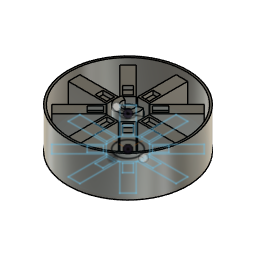
Pill Organiser Archive (Autodesk Fusion 360 design; units mm, degrees)
Autodesk Fusion 360 part; units mm, degrees
note: some values were not read from the file. Set by a fixed rule: which sketch regions a step uses.
sketch "Pill Organiser" plane through (0, 0, 0) normal (0, 0, 1) x (1, 0, 0)
  circle A0 centre (0, 0) radius 150
  dimension "d9" = 300
  constraint coincident A0.centre origin
  measures "d9" diameter of A0
extrude "Extrude2" add sketch "Pill Organiser" along normal blind 30
shell "Shell2" thickness 5 outward yes removed faces 1 at (37.2111, 41.4608, 30)
sketch "Compartment Mounts" plane through (0, 0, 0) normal (0, 0, 1) x (-1, 0, 0)
  circle A0 centre (0, 0) radius 150
  circle A1 centre (0, 0) radius 30
  line L0 (15, -140) -> (-15, -140)
  line L1 (-15, -140) -> (-15, -40)
  line L2 (-15, -40) -> (15, -40)
  line L3 (15, -40) -> (15, -140)
  line L4 (0, -40) -> (0, 0) construction
  line L5 (0, 0) -> (0, 40) construction
  line L6 (-15, 40) -> (-15, 140)
  line L7 (15, 40) -> (-15, 40)
  line L8 (15, 140) -> (15, 40)
  line L9 (-15, 140) -> (15, 140)
  line L10 (140, 15) -> (140, -15)
  line L11 (140, -15) -> (40, -15)
  line L12 (40, -15) -> (40, 15)
  line L13 (40, 15) -> (140, 15)
  line L14 (0, 0) -> (40, 0) construction
  line L15 (0, 0) -> (-40, 0) construction
  line L16 (-140, 15) -> (-40, 15)
  line L17 (-40, 15) -> (-40, -15)
  line L18 (-140, -15) -> (-140, 15)
  line L19 (-40, -15) -> (-140, -15)
  line L20 (10, -45) -> (-10, -45)
  line L21 (-10, -45) -> (-10, -75)
  line L22 (-10, -75) -> (10, -75)
  line L23 (10, -75) -> (10, -45)
  line L24 (-45, -10) -> (-75, -10)
  line L25 (-75, -10) -> (-75, 10)
  line L26 (-75, 10) -> (-45, 10)
  line L27 (-45, 10) -> (-45, -10)
  line L28 (10, 45) -> (-10, 45)
  line L29 (-10, 45) -> (-10, 75)
  line L30 (-10, 75) -> (10, 75)
  line L31 (10, 75) -> (10, 45)
  line L32 (75, -10) -> (45, -10)
  line L33 (45, -10) -> (45, 10)
  line L34 (45, 10) -> (75, 10)
  line L35 (75, 10) -> (75, -10)
  line L36 (-109.6016, -88.3883) -> (-38.8909, -17.6777)
  line L37 (-38.8909, -17.6777) -> (-17.6777, -38.8909)
  line L38 (-17.6777, -38.8909) -> (-88.3883, -109.6016)
  line L39 (-88.3883, -109.6016) -> (-109.6016, -88.3883)
  line L40 (-38.8909, -24.7487) -> (-24.7487, -38.8909)
  line L41 (-24.7487, -38.8909) -> (-45.9619, -60.1041)
  line L42 (-60.1041, -45.9619) -> (-38.8909, -24.7487)
  line L43 (-45.9619, -60.1041) -> (-60.1041, -45.9619)
  line L44 (38.8909, -17.6777) -> (109.6016, -88.3883)
  line L45 (109.6016, -88.3883) -> (88.3883, -109.6016)
  line L46 (17.6777, -38.8909) -> (38.8909, -17.6777)
  line L47 (88.3883, -109.6016) -> (17.6777, -38.8909)
  line L48 (38.8909, -24.7487) -> (24.7487, -38.8909)
  line L49 (24.7487, -38.8909) -> (45.9619, -60.1041)
  line L50 (60.1041, -45.9619) -> (38.8909, -24.7487)
  line L51 (45.9619, -60.1041) -> (60.1041, -45.9619)
  line L52 (-88.3883, 109.6016) -> (-17.6777, 38.8909)
  line L53 (-17.6777, 38.8909) -> (-38.8909, 17.6777)
  line L54 (-109.6016, 88.3883) -> (-88.3883, 109.6016)
  line L55 (-38.8909, 17.6777) -> (-109.6016, 88.3883)
  line L56 (-45.9619, 60.1041) -> (-24.7487, 38.8909)
  line L57 (-24.7487, 38.8909) -> (-38.8909, 24.7487)
  line L58 (-60.1041, 45.9619) -> (-45.9619, 60.1041)
  line L59 (-38.8909, 24.7487) -> (-60.1041, 45.9619)
  line L60 (109.6016, 88.3883) -> (38.8909, 17.6777)
  line L61 (38.8909, 17.6777) -> (17.6777, 38.8909)
  line L62 (88.3883, 109.6016) -> (109.6016, 88.3883)
  line L63 (17.6777, 38.8909) -> (88.3883, 109.6016)
  line L64 (38.8909, 24.7487) -> (24.7487, 38.8909)
  line L65 (24.7487, 38.8909) -> (45.9619, 60.1041)
  line L66 (60.1041, 45.9619) -> (38.8909, 24.7487)
  line L67 (45.9619, 60.1041) -> (60.1041, 45.9619)
  dimension "d93" = 60
  dimension "d96" = 30
  dimension "d97" = 100
  dimension "d106" = 40
  dimension "d107" = 30
  dimension "d108" = 100
  dimension "d110" = 100
  dimension "d111" = 30
  dimension "d112" = 100
  dimension "d113" = 30
  dimension "d114" = 20
  dimension "d115" = 30
  dimension "d116" = 30
  dimension "d117" = 20
  dimension "d118" = 20
  dimension "d119" = 30
  dimension "d120" = 30
  dimension "d121" = 100
  dimension "d122" = 30
  dimension "d123" = 100
  dimension "d124" = 100
  dimension "d125" = 30
  dimension "d126" = 100
  dimension "d127" = 30
  dimension "d128" = 20
  dimension "d129" = 30
  dimension "d130" = 30
  dimension "d131" = 20
  dimension "d132" = 20
  dimension "d133" = 30
  constraint coincident A0.centre A1.centre
  constraint horizontal L0
  constraint vertical L1
  constraint horizontal L2
  constraint vertical L3
  constraint midpoint L2 L4.start
  constraint perpendicular L2 L5
  constraint horizontal L7
  constraint vertical L6
  constraint horizontal L9
  constraint vertical L8
  constraint horizontal L11
  constraint vertical L12
  constraint horizontal L13
  constraint vertical L10
  constraint midpoint L12 L14.end
  constraint perpendicular L5 L15
  constraint horizontal L19
  constraint vertical L18
  constraint horizontal L16
  constraint vertical L17
  constraint horizontal L20
  constraint vertical L21
  constraint horizontal L22
  constraint vertical L23
  constraint horizontal L24
  constraint vertical L25
  constraint horizontal L26
  constraint vertical L27
  constraint horizontal L28
  constraint vertical L29
  constraint horizontal L30
  constraint vertical L31
  constraint horizontal L32
  constraint vertical L33
  constraint horizontal L34
  constraint vertical L35
  measures "d93" diameter of A1
  measures "d96" distance of L0.start L0.end
  measures "d97" distance of L0.start L2.end
  measures "d106" distance of A0.centre L5.end
  measures "d107" distance of L6.start L7.start
  measures "d108" distance of L8.start L7.start
  measures "d110" distance of L11.end L10.end
  measures "d111" distance of L10.start L10.end
  measures "d112" distance of L18.start L17.end
  measures "d113" distance of L17.end L16.end
  measures "d114" distance of L20.start L20.end
  measures "d115" distance of L20.start L22.end
  measures "d116" distance of L24.start L24.end
  measures "d117" distance of L24.start L26.end
  measures "d118" distance of L28.start L28.end
  measures "d119" distance of L28.start L30.end
  measures "d120" distance of L45.end L44.end
  measures "d121" distance of L44.start L44.end
  measures "d122" distance of L53.end L52.end
  measures "d123" distance of L52.start L52.end
  measures "d124" distance of L60.end L60.start
  measures "d125" distance of L60.start L62.start
  measures "d126" distance of L38.end L37.end
  measures "d127" distance of L36.end L37.end
  measures "d128" distance of L48.start L48.end
  measures "d129" distance of L48.start L50.start
  measures "d130" distance of L40.end L41.end
  measures "d131" distance of L40.end L40.start
  measures "d132" distance of L56.end L57.end
  measures "d133" distance of L56.end L56.start
ref_plane "WorkPlane1" through (32, 0, 0) normal (1, 0, 0) x (0, 1, 0)
ref_plane "WorkPlane2" through (32, 0, 0) normal (1, 0, 0) x (0, 1, 0)
sketch "Motor Stand" plane through (0, 0, 0) normal (0, 0, 1) x (1, 0, 0)
  circle A0 centre (0, 0) radius 30
  dimension "d74" = 60
  constraint coincident A0.centre origin
  measures "d74" diameter of A0
extrude "Extrude9" add sketch "Motor Stand" along normal blind 80
sketch "Motor Holder" plane through (0, 0, 80) normal (0, 0, 1) x (-1, 0, 0)
  circle A0 centre (0, 0) radius 30
  line L0 (0, 0) -> (27.1892, -12.6785) construction
  line L1 (0, 0) -> (30, 0) construction
  line L2 (0, 0) -> (-27.1892, -12.6785) construction
  line L3 (0, 0) -> (30, 0) construction
  arc A1 (14.5009, -6.7619) -> (-14.5009, -6.7619) centre (0, 0) ccw
  line L4 (0, 0) -> (-27.1892, -12.6785)
  line L5 (0, 0) -> (27.1892, -12.6785)
  dimension "d80" = 32
  dimension "d81" = 25
  dimension "d82" = 155
  constraint concentric A0 A1
  constraint horizontal L1
  constraint coincident A0.centre L0.start
  constraint horizontal L3
  constraint coincident L2 A1.end
  constraint coincident L0 A1.start
  constraint parallel L0 L5
  measures "d80" diameter of A1
  measures "d81" angle of L0 L1
  measures "d82" angle of L2 L3
extrude "Extrude10" add sketch "Motor Holder" along normal blind 20 contours A0 A1 L4 L5
extrude "Extrude11" cut 1 faces at (148.2395, 37.6673, 30) along direction (0, 0, -1) blind 10
extrude "Extrude12" cut 1 faces at (148.2395, 37.6673, 20) along direction (0, 0, -1) blind 10
extrude "Extrude13" add 1 faces at (148.2395, 37.6673, 10) along direction (0, 0, 1) blind 90
ref_plane "WorkPlane6" through (0, 0, 12.125) normal (-0.707107, 0.707107, 0) x (0, 0, 1)
extrude "Extrude14" add sketch "Compartment Mounts" along normal blind 80 contours L20 L21 L22 L23 | L24 L25 L26 L27 | L28 L29 L30 L31 | L32 L33 L34 L35 | L40 L41 L42 L43 | L48 L49 L50 L51 | L56 L57 L58 L59 | L64 L65 L66 L67
extrude "Extrude15" add sketch "Compartment Mounts" along normal blind 90 contours L0 L1 L2 L3 | L6 L7 L8 L9 | L10 L11 L12 L13 | L16 L17 L18 L19 | L36 L37 L38 L39 | L44 L45 L46 L47 | L52 L53 L54 L55 | L60 L61 L62 L63
